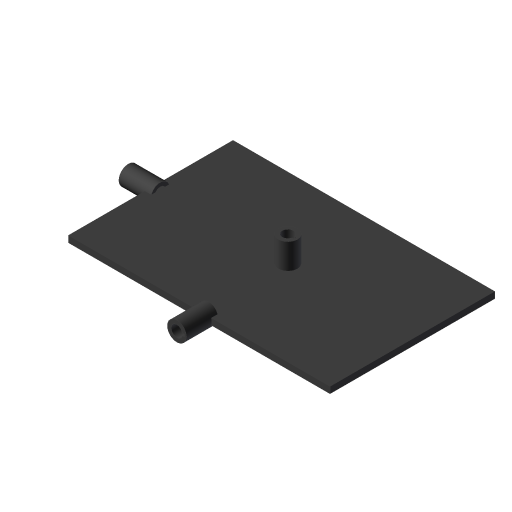
# Autodesk Inventor part: GroundCorrected
Saved by Autodesk Inventor 2023.4 (Build 274418000, 418)
## iProperties
Created: 2024-03-05
Part Number: GroundCorrected
Material: Generic
Document SubType Name: Modeling
Designer: josep
Density: 1 g/cm^3
Appearance: Default
Author: josep
Autodesk Inventor part; units mm, degrees
ref_plane "YZ Plane" through (0, 0, 0) normal (1, 0, 0) x (0, 1, 0)
ref_plane "XZ Plane" through (0, 0, 0) normal (0, 1, 0) x (-1, 0, 0)
ref_plane "XY Plane" through (0, 0, 0) normal (0, 0, 1) x (1, 0, 0)
sketch "Sketch1" plane through (0, 0, 0) normal (0, 1, 0) x (-1, 0, 0)
  line L0 (102.5, 64.5) -> (-102.5, 64.5)
  line L1 (-102.5, 64.5) -> (-102.5, -64.5)
  line L2 (-102.5, -64.5) -> (102.5, -64.5)
  line L3 (102.5, -64.5) -> (102.5, 64.5)
  line L4 (0, 64.5) -> (0, -64.5)
  line L5 (102.5, 0) -> (-102.5, 0)
  point P0 (0, 0)
  dimension "d0" = 129
  dimension "d1" = 205
  dimension "d2" = 0
  dimension "d3" = 0
  constraints: 12 end point, 4 midpoint, 2 parallel, 1 horizontal, 1 perpendicular, 1 vertical
  measures "d0" distance of L2.end L0.start
  measures "d1" distance of L1.end L2.end
  measures "d2" vertical distance of L5.start point (0, 0)
  measures "d3" horizontal distance of L4.end point (0, 0)
extrude "Extrusion1" add sketch "Sketch1" along normal blind 5
sketch "Sketch2" plane through (0, 5, 0) normal (0, 1, 0) x (1, 0, 0)
  circle A0 centre (2.5, 2.5) radius 4.5
  circle A1 centre (2.5, 2.5) radius 6
  circle A2 centre (2.5, 2.5) radius 7.5
  circle A3 centre (2.5, 2.5) radius 2.35
  line L0 (6.8875, 3.5) -> (9.933, 3.5)
  line L1 (6.8875, 1.5) -> (9.933, 1.5)
  line L2 (-102.5, 64.5) -> (-102.5, -64.5) projected
  line L3 (102.5, -64.5) -> (102.5, 64.5) projected
  line L4 (-102.5, -64.5) -> (102.5, -64.5)
  line L5 (102.5, -64.5) -> (102.5, 64.5)
  line L6 (102.5, 64.5) -> (-102.5, 64.5)
  line L7 (-102.5, 64.5) -> (-102.5, -64.5)
  line L8 (-102.5, -64.5) -> (102.5, -64.5) projected
  point P0 (0, -64.5)
  point P1 (8.4161, 3.5)
  point P2 (8.4161, 1.5)
  point P3 (-102.5, 0)
  dimension "d18" = 9
  dimension "d19" = 12
  dimension "d20" = 15
  dimension "d21" = 4.7
  dimension "d22" = 1
  dimension "d23" = 1
  dimension "d26" = 0
  dimension "d40" = 67
  dimension "d41" = 105
  constraints: 12 end point, 4 centre point, 4 point on circle, 3 coincident, 3 parallel, 2 horizontal, 2 midpoint, 1 perpendicular
  measures "d18" diameter of A0
  measures "d19" diameter of A1
  measures "d20" diameter of A2
  measures "d21" diameter of A3
  measures "d22" vertical distance of point (2.5, 2.5) L0.end
  measures "d23" vertical distance of point (2.5, 2.5) L1.end
  measures "d26" distance of A0.centre point (2.5, 2.5)
  measures "d40" vertical distance of L2.end point (2.5, 2.5)
  measures "d41" horizontal distance of L2.end point (2.5, 2.5)
extrude "Extrusion2" add sketch "Sketch2" along normal blind 20 contours A0 L1 A1 L0 | L0 A2 L1 A1 | A1 L1 A2 L0 picked at (-2.8948, 1.6483)
sketch "Sketch3" plane through (-102.5, 0, 64.5) normal (0, 0, 1) x (1, 0, 0)
  circle A0 centre (105, 2.5) radius 4.5
  circle A1 centre (105, 2.5) radius 6
  circle A2 centre (105, 2.5) radius 7.5
  circle A3 centre (105, 2.5) radius 2.35
  line L0 (109.3875, 3.5) -> (112.433, 3.5)
  line L1 (109.3875, 1.5) -> (112.433, 1.5)
  line L2 (0, 0) -> (0, 5) projected
  point P0 (102.5, 0)
  point P1 (0, 2.5)
  point P2 (110.9161, 3.5)
  point P3 (110.9161, 1.5)
  dimension "d30" = 9
  dimension "d31" = 12
  dimension "d32" = 15
  dimension "d33" = 4.7
  dimension "d34" = 1
  dimension "d35" = 1
  dimension "d36" = 0
  dimension "d37" = 105
  dimension "d38" = 0
  constraints: 4 centre point, 4 end point, 4 point on circle, 3 coincident, 1 horizontal, 1 midpoint, 1 parallel
  measures "d30" diameter of A0
  measures "d31" diameter of A1
  measures "d32" diameter of A2
  measures "d33" diameter of A3
  measures "d34" vertical distance of point (105, 2.5) L0.end
  measures "d35" vertical distance of point (105, 2.5) L1.end
  measures "d36" distance of A0.centre point (105, 2.5)
  measures "d37" distance from line of L2 A3.centre
  measures "d38" vertical distance of point (0, 2.5) A3.centre
extrude "Extrusion3" add sketch "Sketch3" along normal blind 20 and the other way blind 5 contours A0 L1 A1 L0 | L0 A2 L1 A1 | A1 L1 A2 L0 picked at (99.6052, 1.6483)
sketch "Sketch4" plane through (-102.5, 0, -64.5) normal (-1, 0, 0) x (0, 0, 1)
  circle A0 centre (62, 2.5) radius 4.5
  circle A1 centre (62, 2.5) radius 6
  circle A2 centre (62, 2.5) radius 7.5
  circle A3 centre (62, 2.5) radius 2.35
  line L0 (66.3875, 3.5) -> (69.433, 3.5)
  line L1 (66.3875, 1.5) -> (69.433, 1.5)
  line L2 (129, 0) -> (129, 5) projected
  point P0 (64.5, 0)
  point P1 (129, 2.5)
  point P2 (67.9161, 3.5)
  point P3 (67.9161, 1.5)
  dimension "d46" = 9
  dimension "d47" = 12
  dimension "d48" = 15
  dimension "d49" = 4.7
  dimension "d50" = 1
  dimension "d51" = 1
  dimension "d52" = 0
  dimension "d53" = 0
  dimension "d54" = 67
  constraints: 4 centre point, 4 end point, 4 point on circle, 3 coincident, 1 horizontal, 1 midpoint, 1 parallel
  measures "d46" diameter of A0
  measures "d47" diameter of A1
  measures "d48" diameter of A2
  measures "d49" diameter of A3
  measures "d50" vertical distance of point (62, 2.5) L0.end
  measures "d51" vertical distance of point (62, 2.5) L1.end
  measures "d52" distance of A0.centre point (62, 2.5)
  measures "d53" vertical distance of point (129, 2.5) A3.centre
  measures "d54" distance from line of L2 A3.centre
extrude "Extrusion4" add sketch "Sketch4" along normal blind 20 and the other way blind 5 contours A0 L1 A1 L0 | L0 A2 L1 A1 | A1 L1 A2 L0 picked at (56.6052, 1.6483)
body "Solid1"
